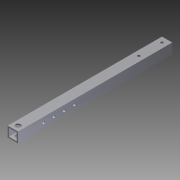
# Autodesk Inventor part: bambar 12 in
Saved by Autodesk Inventor 2011 SP1 (Build 150282100, 282)
## iProperties
Created: 2012-01-18
Part Number: bambar 12 in
Document SubType Name: Modeling
Designer: Christopher
Density: 1 g/cm^3
Author: Christopher
Autodesk Inventor part; units mm, degrees
ref_plane "YZ Plane" through (0, 0, 0) normal (1, 0, 0) x (0, 1, 0)
ref_plane "XZ Plane" through (0, 0, 0) normal (0, 1, 0) x (-1, 0, 0)
ref_plane "XY Plane" through (0, 0, 0) normal (0, 0, 1) x (1, 0, 0)
sketch "Sketch1" plane through (0, 0, 0) normal (0, 0, 1) x (1, 0, 0)
  line L0 (0, 0) -> (25.4, 0)
  line L1 (25.4, 0) -> (25.4, 25.4)
  line L2 (25.4, 25.4) -> (0, 25.4)
  line L3 (0, 25.4) -> (0, 0)
  line L4 (3.175, 3.175) -> (22.225, 3.175)
  line L5 (22.225, 3.175) -> (22.225, 22.225)
  line L6 (22.225, 22.225) -> (3.175, 22.225)
  line L7 (3.175, 22.225) -> (3.175, 3.175)
  dimension "d0" = 25.4
  dimension "d1" = 25.4
  dimension "d2" = 3.175
  constraints: 16 end point, 4 parallel, 2 perpendicular, 1 horizontal, 3 other
  measures "d0" distance of L1.end L2.end
  measures "d1" distance of L0.end L1.end
  measures "d2" distance between parallel lines of L3 L7
extrude "Extrusion1" add sketch "Sketch1" against normal blind 381
sketch "Sketch2" plane through (0, 25.4, 0) normal (0, 1, 0) x (1, 0, 0)
  line L0 (25.4, 381) -> (0, 381) projected
  line L1 (25.4, 0) -> (0, 0) projected
  line L2 (25.4, 0) -> (25.4, 381) projected
  point P0 (12.7, 368.3)
  point P1 (12.7, 311.15)
  point P2 (12.7, 12.7)
  dimension "d5" = 12.7
  dimension "d6" = 57.15
  dimension "d25" = 12.7
  dimension "d26" = 12.7
  measures "d5" distance from line of L0 point (12.7, 368.3)
  measures "d6" distance of point (12.7, 368.3) point (12.7, 311.15)
  measures "d25" distance from line of L2 point (12.7, 12.7)
  measures "d26" distance from line of L1 point (12.7, 12.7)
hole "Hole1" at (12.7, 25.4, -368.3) at (12.7, 25.4, -311.15) direction (0, -1, 0) diameter 6.35 depth 25.4 tip angle 118
sketch "Sketch3" plane through (25.4, 0, 0) normal (1, 0, 0) x (0, 0, -1)
  line L0 (0, 0) -> (0, 25.4) projected
  point P0 (63.5, 12.7)
  point P1 (0, 12.7)
  point P2 (88.9, 12.7)
  point P3 (114.3, 12.7)
  point P4 (0, 12.7)
  point P5 (139.7, 12.7)
  dimension "d14" = 63.5
  dimension "d15" = 25.4
  dimension "d16" = 25.4
  dimension "d24" = 139.7
  constraints: 4 horizontal alignment, 2 midpoint
  measures "d14" distance from line of point (63.5, 12.7) L0
  measures "d15" distance of point (63.5, 12.7) point (88.9, 12.7)
  measures "d16" distance of point (88.9, 12.7) point (114.3, 12.7)
  measures "d24" distance from line of L0 point (139.7, 12.7)
hole "Hole2" at (25.4, 12.7, -63.5) at (25.4, 12.7, -88.9) at (25.4, 12.7, -114.3) at (25.4, 12.7, -139.7) direction (-1, 0, 0) diameter 6.35 depth 25.4 tip angle 118
hole "Hole3" at (12.7, 25.4, -12.7) direction (0, -1, 0) diameter 12.7 depth 25.4 tip angle 118
body "Solid1"
